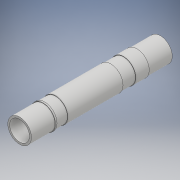
# Autodesk Inventor part: Axe manivelles
Saved by Autodesk Inventor 2018.1 (Build 221171000, 171)
## iProperties
Created: 2022-05-13
Part Number: Axe manivelles
Material: Generic
Document SubType Name: Modeling
Designer: Bureau
Density: 1 g/cm^3
Appearance: Default
Author: Bureau
Autodesk Inventor part; units mm, degrees
ref_plane "YZ Plane" through (0, 0, 0) normal (1, 0, 0) x (0, 1, 0)
ref_plane "XZ Plane" through (0, 0, 0) normal (0, 1, 0) x (-1, 0, 0)
ref_plane "XY Plane" through (0, 0, 0) normal (0, 0, 1) x (1, 0, 0)
sketch "Sketch1" plane through (0, 0, 0) normal (0, 0, 1) x (1, 0, 0)
  line L0 (0, 0) -> (10, 0)
  line L1 (10, 0) -> (12, 0)
  line L2 (10, 0) -> (10, 142.5)
  line L3 (0, 0) -> (0, 30)
  line L4 (12, 0) -> (12, 23.8)
  line L5 (12, 23.8) -> (12.5, 23.8)
  line L6 (12.5, 23.8) -> (12.5, 25.4)
  line L7 (12.5, 25.4) -> (12, 25.4)
  line L8 (12, 25.4) -> (12, 36.4)
  line L9 (12, 36.4) -> (12.5, 36.4)
  line L10 (12.5, 118.7) -> (12, 118.7)
  line L11 (12, 118.7) -> (12, 142.5)
  line L12 (12, 142.5) -> (10, 142.5)
  line L13 (12.5, 118.7) -> (12.5, 105.2)
  line L14 (12.5, 105.2) -> (12, 105.2)
  line L15 (12, 105.2) -> (12, 92.2)
  line L16 (12, 92.2) -> (12.5, 92.2)
  line L17 (12.5, 36.4) -> (12.5, 92.2)
  line L18 (12.5, 105.2) -> (12.5, 118.7)
  dimension "d0" = 10
  dimension "d1" = 2
  dimension "d2" = 142.5
  dimension "d4" = 30
  dimension "d6" = 23.8
  dimension "d7" = 0.5
  dimension "d8" = 1.6
  dimension "d9" = 11
  dimension "d10" = 90
  dimension "d11" = 0.5
  dimension "d12" = 82.3
  dimension "d13" = 13.5
  dimension "d14" = 0.5
  dimension "d15" = 13
  constraints: 38 end point, 9 perpendicular, 6 point on line, 4 vertical, 1 horizontal
  measures "d0" distance of L0.start L0.end
  measures "d1" distance of L0.end L1.end
  measures "d2" distance of L0.end L2.end
  measures "d4" distance of L0.start L3.end
  measures "d6" distance of L1.end L4.end
  measures "d7" distance of L4.end L5.end
  measures "d8" distance of L5.end L6.end
  measures "d9" distance of L7.end L8.end
  measures "d10" angle of L7 L8
  measures "d11" distance of L8.end L9.end
  measures "d12" distance of L9.end L10.start
  measures "d13" distance of L10.start L13.end
  measures "d14" distance of L13.end L14.end
  measures "d15" distance of L14.end L15.end
revolve "Revolution1" add sketch "Sketch1" angle 360 about axis through (0, 0, 0) along (0, 1, 0)
body "Solid1"
